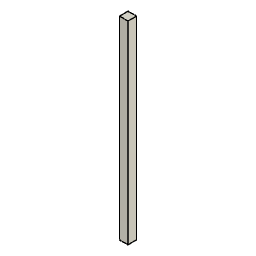
back_panel_support_left (Autodesk Fusion 360 design; units mm, degrees)
Autodesk Fusion 360 part; units mm, degrees
sketch "Back Panel Support Left " plane through (0, 0, 0) normal (1, 0, 0) x (0, 1, 0)
  line L0 (0, 0) -> (21, 0)
  line L1 (21, 0) -> (21, 478.576)
  line L2 (21, 478.576) -> (0, 478.576)
  line L3 (0, 478.576) -> (0, 0)
  dimension "d1" = 478.576
  dimension "d2" = 21
  constraint horizontal L0
  constraint vertical L1
  constraint horizontal L2
  constraint vertical L3
  constraint coincident L0.start L3.end
  measures "d1" distance of L0.end L1.end
  measures "d2" distance of L0.start L0.end
extrude "Extrude1" add sketch "Back Panel Support Left " along normal blind 21
named bodies: "Back Panel Support Left"
